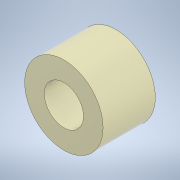
# Autodesk Inventor part: PEAKスペーサーm3中空-4
Saved by Autodesk Inventor 2020.2 (Build 242310000, 310)
## iProperties
Created: 2020-05-11
Part Number: PEAKスペーサーm3中空-4
Material: PAEK 樹脂
Document SubType Name: Modeling
Designer: mozar
Density: 1.32 g/cm^3
Appearance: 滑らか - 灰色
Mass: 0.0839748 g
Surface Area: 1.27235 cm^2
Volume: 0.0636173 cm^3
Author: mozar
Autodesk Inventor part; units mm, degrees
ref_plane "YZ Plane" through (0, 0, 0) normal (1, 0, 0) x (0, 1, 0)
ref_plane "XZ Plane" through (0, 0, 0) normal (0, 1, 0) x (-1, 0, 0)
ref_plane "XY Plane" through (0, 0, 0) normal (0, 0, 1) x (1, 0, 0)
sketch "スケッチ1" plane through (0, 0, 0) normal (0, 0, 1) x (1, 0, 0)
  circle A0 centre (0, 0) radius 3
  circle A1 centre (0, 0) radius 1.5
  dimension "d0" = 6
  dimension "d1" = 3
  constraints: 2 centre point, 2 coincident
  measures "d0" diameter of A0
  measures "d1" diameter of A1
extrude "押し出し1" add sketch "スケッチ1" against normal blind 4
